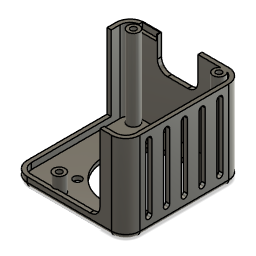
Fan Shroud (Autodesk Fusion 360 design; units mm, degrees)
Autodesk Fusion 360 part; units mm, degrees
sketch "Sketch1" plane through (0, 0, 0) normal (0, 1, 0) x (1, 0, 0)
  circle A0 centre (0, 0) radius 19
  circle A1 centre (-16, 16) radius 2
  circle A2 centre (16, 16) radius 2
  circle A3 centre (16, -16) radius 2
  circle A4 centre (-16, -16) radius 2
  line L0 (-26.4, 25.4) -> (15.2, 25.4)
  line L1 (20.2, 20.4) -> (20.2, -23.4)
  line L2 (15.2, -28.4) -> (-26.4, -28.4)
  line L3 (-31.4, -23.4) -> (-31.4, 20.4)
  line L4 (9.5, -30.4) -> (9.5, -28.4)
  line L5 (-31.4, 16) -> (-33.4, 16)
  arc A5 (15.2, -28.4) -> (20.2, -23.4) centre (15.2, -23.4) ccw
  arc A6 (20.2, 20.4) -> (15.2, 25.4) centre (15.2, 20.4) ccw
  arc A7 (-26.4, 25.4) -> (-31.4, 20.4) centre (-26.4, 20.4) ccw
  arc A8 (-31.4, -23.4) -> (-26.4, -28.4) centre (-26.4, -23.4) ccw
  line L6 (15.2, -30.4) -> (-26.4, -30.4)
  arc A9 (-33.4, -23.4) -> (-26.4, -30.4) centre (-26.4, -23.4) ccw
  line L7 (-33.4, -23.4) -> (-33.4, 20.4)
  arc A10 (-26.4, 27.4) -> (-33.4, 20.4) centre (-26.4, 20.4) ccw
  line L8 (-26.4, 27.4) -> (15.2, 27.4)
  arc A11 (22.2, 20.4) -> (15.2, 27.4) centre (15.2, 20.4) ccw
  line L9 (22.2, 20.4) -> (22.2, -23.4)
  arc A12 (15.2, -30.4) -> (22.2, -23.4) centre (15.2, -23.4) ccw
  dimension "d3" = 38
  dimension "d4" = 4
  dimension "d5" = 4
  dimension "d6" = 4
  dimension "d7" = 4
  dimension "d8" = 32
  dimension "d9" = 32
  dimension "d10" = 16
  dimension "d11" = 16
  dimension "d33" = 20.2
  dimension "d46" = 25.4
  dimension "d47" = 28.4
  dimension "d55" = 31.4
  dimension "d56" = 9.5
  dimension "d81" = 5
  dimension "d82" = 2
  dimension "d138" = 5
  dimension "d139" = 5
  dimension "d140" = 5
  dimension "d141" = 16
  constraint coincident A0.centre origin
  constraint vertical A1.centre A4.centre
  constraint horizontal A1.centre A2.centre
  constraint vertical A2.centre A3.centre
  constraint horizontal A3.centre A4.centre
  constraint horizontal L0
  constraint vertical L1
  constraint horizontal L2
  constraint vertical L3
  constraint coincident L2 L4.end
  constraint perpendicular L2 L4
  constraint coincident L3 L5.start
  constraint tangent L2 A5
  constraint tangent L1 A5
  constraint tangent L0 A6
  constraint tangent L1 A6
  constraint tangent L0 A7
  constraint tangent L3 A7
  constraint tangent L3 A8
  constraint tangent L2 A8
  constraint coincident L4.start L6
  constraint horizontal L5
  constraint coincident L5.end L7
  measures "d3" diameter of A0
  measures "d4" diameter of A1
  measures "d5" diameter of A2
  measures "d6" diameter of A3
  measures "d7" diameter of A4
  measures "d8" distance of A1.centre A4.centre
  measures "d9" distance of A3.centre A4.centre
  measures "d10" horizontal distance of A0.centre A4.centre
  measures "d11" vertical distance of A0.centre A4.centre
  measures "d33" distance of A0.centre L1
  measures "d46" distance of A0.centre L0
  measures "d47" distance of A0.centre L2
  measures "d55" distance of A0.centre L3
  measures "d56" distance of A0.centre L4
  measures "d81" radius of A8
  measures "d138" radius of A7
  measures "d139" radius of A6
  measures "d140" radius of A5
  measures "d141" distance of A0.centre L5
extrude "Extrude1" add sketch "Sketch1" along normal blind 2 contours L0 L1 L2 L3 A5 A6 A7 A8 makes body 1
sketch "Sketch2" plane through (0, 2, 0) normal (0, 1, 0) x (-1, 0, 0)
  circle A0 centre (-16, -16) radius 2
  circle A1 centre (0, 0) radius 19
  circle A2 centre (16, 16) radius 2
  circle A3 centre (-16, 16) radius 2
  circle A4 centre (16, -16) radius 2
  circle A5 centre (-14.75, -23) radius 1.4
  circle A6 centre (26.4, -22) radius 1.4
  circle A7 centre (15, 26) radius 1.4
  line L0 (31.4, -20.4) -> (31.4, 23.4)
  line L1 (26.4, 28.4) -> (-15.2, 28.4)
  line L2 (-20.2, 23.4) -> (-20.2, -20.4)
  line L3 (-15.2, -25.4) -> (26.4, -25.4)
  arc A8 (-15.2, 28.4) -> (-20.2, 23.4) centre (-15.2, 23.4) ccw
  arc A9 (-20.2, -20.4) -> (-15.2, -25.4) centre (-15.2, -20.4) ccw
  arc A10 (26.4, -25.4) -> (31.4, -20.4) centre (26.4, -20.4) ccw
  arc A11 (31.4, 23.4) -> (26.4, 28.4) centre (26.4, 23.4) ccw
  circle A12 centre (26.4, -22) radius 2.9
  circle A13 centre (-14.75, -23) radius 2.9
  circle A14 centre (15, 26) radius 2.9
  line L4 (20.2, -20.2) -> (-20.2, -20.2)
  line L5 (-20.2, -20.2) -> (-20.2, 20.2)
  line L6 (-20.2, 20.2) -> (20.2, 20.2)
  line L7 (20.2, 20.2) -> (20.2, -20.2)
  line L8 (20.2, -20.2) -> (-20.2, 20.2) construction
  line L9 (-20.2, -20.2) -> (20.2, 20.2) construction
  dimension "d14" = 2.8
  dimension "d16" = 23
  dimension "d17" = 2.8
  dimension "d19" = 22
  dimension "d26" = 2.8
  dimension "d57" = 26.4
  dimension "d58" = 14.75
  dimension "d88" = 1.5
  dimension "d89" = 1.5
  dimension "d90" = 1.5
  dimension "d91" = 40.4
  dimension "d92" = 40.4
  dimension "d142" = 48
  dimension "d143" = 11.4
  constraint horizontal L4
  constraint perpendicular L4 L5
  constraint parallel L4 L6
  constraint parallel L5 L7
  constraint coincident L8 A1.centre
  constraint coincident L9 A1.centre
  constraint coincident A1.centre origin
  measures "d14" diameter of A5
  measures "d16" vertical distance of A1.centre A5.centre
  measures "d17" diameter of A6
  measures "d19" vertical distance of A1.centre A6.centre
  measures "d26" diameter of A7
  measures "d57" horizontal distance of A1.centre A6.centre
  measures "d58" horizontal distance of A1.centre A5.centre
  measures "d91" distance of L5.end L6.end
  measures "d92" distance of L4.end L5.end
  measures "d142" vertical distance of A6.centre A7.centre
  measures "d143" horizontal distance of A6.centre A7.centre
extrude "Extrude2" add sketch "Sketch2" along normal blind 41.5 contours L3 A9 A13 | L3 A9 A13 L4 | A13 L4 bodies 1
extrude "Extrude3" add sketch "Sketch2" along normal blind 40 contours A12 bodies 1
extrude "Extrude4" add sketch "Sketch2" along normal blind 8.6 contours L1 A14 | L1 A14 bodies 1
extrude "Extrude6" add sketch "Sketch1" along normal blind 43.5 contours L0 L1 L2 L3 L4 L5 A5 A6 A7 L6 L7 A10 L8 A11 L9 A12 bodies 1
extrude "Extrude7" add sketch "Sketch1" along normal blind 5 separate body contours L2 L3 L4 L5 A8 L6 A9 L7 makes body 2
sketch "Sketch3" plane through (0, 0, -27.4) normal (0, 0, -1) x (-1, 0, 0)
  line L0 (-15.2, 0) -> (26.4, 0)
  line L1 (26.4, 0) -> (26.4, 43.5)
  line L2 (26.4, 43.5) -> (-15.2, 43.5)
  line L3 (-15.2, 43.5) -> (-15.2, 0)
  line L4 (-2, 43.5) -> (18, 43.5)
  line L5 (18, 43.5) -> (18, 31.5)
  line L6 (13, 26.5) -> (3, 26.5)
  line L7 (-2, 31.5) -> (-2, 43.5)
  arc A0 (13, 26.5) -> (18, 31.5) centre (13, 31.5) ccw
  arc A1 (-2, 31.5) -> (3, 26.5) centre (3, 31.5) ccw
  line L8 (-15.2, 0) -> (26.4, 0)
  line L9 (26.4, 0) -> (26.4, 43.5)
  line L10 (26.4, 43.5) -> (-15.2, 43.5)
  line L11 (-15.2, 43.5) -> (-15.2, 0)
  dimension "d67" = 17
  dimension "d68" = 5
  dimension "d144" = 2
  dimension "d145" = 20
  constraint horizontal L4
  constraint perpendicular L4 L5
  constraint parallel L4 L6
  constraint parallel L5 L7
  constraint coincident L2.end L4
  constraint tangent L5 A0
  constraint tangent L6 A0
  constraint tangent L6 A1
  constraint tangent L7 A1
  constraint equal A0 A1
  measures "d67" distance of L4 L6
  measures "d68" radius of A0
  measures "d144" distance of origin L7
  measures "d145" distance of L5 L7
extrude "Extrude8" cut sketch "Sketch3" against normal blind 2 contours L2 L4 L5 L6 L7 A0 A1 L10 bodies 1
combine "Combine1" operation add target body 2 tool bodies 1
fillet "Fillet1" radius 5 1 edges at (9.5, 5, 29.4) on bodies 2
fillet "Fillet2" radius 2.5 8 edges at (-31.3497, 0, 28.3497) (-5.6, 0, 30.4) (20.1497, 0, 28.3497) (22.2, 0, 1.5) (20.1497, 0, -25.3497) (-5.6, 0, -27.4) (-31.3497, 0, -25.3497) (-33.4, 0, 1.5) on bodies 2
sketch "Sketch14" plane through (0, 43.5, 0) normal (0, 1, 0) x (-1, 0, 0)
  line L0 (18, -25.4) -> (18, -27.4)
  line L1 (18, -27.4) -> (26.4, -27.4)
  arc A0 (26.4, -27.4) -> (33.4, -20.4) centre (26.4, -20.4) ccw
  line L2 (33.4, -20.4) -> (33.4, -16)
  line L3 (33.4, -16) -> (31.4, -16)
  line L4 (31.4, -16) -> (31.4, -20.4)
  arc A1 (26.4, -25.4) -> (31.4, -20.4) centre (26.4, -20.4) ccw
  line L5 (26.4, -25.4) -> (18, -25.4)
extrude "Extrude14" cut sketch "Sketch14" against normal blind 1.5 bodies 2
sketch "Sketch17" plane through (0, 42, 0) normal (0, 1, 0) x (-1, 0, 0)
  line L0 (26.4, -25.4) -> (18, -25.4)
  line L1 (18, -27.4) -> (26.4, -27.4)
  arc A0 (26.4, -27.4) -> (33.4, -20.4) centre (26.4, -20.4) ccw
  line L2 (33.4, -20.4) -> (33.4, -16)
  line L3 (33.4, -16) -> (31.4, -16)
  line L4 (31.4, -16) -> (31.4, -20.4)
  arc A1 (26.4, -25.4) -> (31.4, -20.4) centre (26.4, -20.4) ccw
  line L5 (18.4, -27) -> (27, -27)
  line L6 (27, -27) -> (27, -25.3639)
  line L7 (18.4, -25.3639) -> (18.4, -27)
  line L8 (18, -25.4) -> (18, -27.4)
  line L9 (19, -26.5) -> (27, -26.5)
  dimension "d133" = 8.6
  dimension "d134" = 0.4
  dimension "d162" = 0.4
  dimension "d163" = 8
  constraint horizontal L5
  constraint vertical L6
  constraint vertical L7
  constraint coincident A1 L6.end
  constraint perpendicular L7 L9
  measures "d133" distance of L5.start L5.end
  measures "d134" distance of L1 L5
  measures "d162" distance of L7 L8
  measures "d163" distance of L9.start L9.end
extrude "Extrude15" cut sketch "Sketch17" against normal blind 3 contours L0 A1 L5 L6 L7 bodies 2
sketch "Sketch19" plane through (22.2, 0, 0) normal (1, 0, 0) x (0, 0, -1)
  line L0 (-23.4, 2.5) -> (20.4, 2.5)
  line L1 (20.4, 2.5) -> (20.4, 43.5)
  line L2 (20.4, 43.5) -> (-23.4, 43.5)
  line L3 (-23.4, 43.5) -> (-23.4, 2.5)
  line L4 (-20.52, 6.88) -> (-20.52, 39.12)
  line L5 (-17.52, 39.12) -> (-17.52, 6.88)
  line L6 (-17.52, 5.88) -> (-20.52, 40.62) construction
  line L7 (-20.52, 5.88) -> (-17.52, 40.62) construction
  arc A0 (-19.02, 40.62) -> (-20.52, 39.12) centre (-19.02, 39.12) ccw
  arc A1 (-17.52, 39.12) -> (-19.02, 40.62) centre (-19.02, 39.12) ccw
  arc A2 (-19.0138, 5.38) -> (-17.52, 6.88) centre (-19.02, 6.88) ccw
  arc A3 (-20.52, 6.88) -> (-19.0138, 5.38) centre (-19.02, 6.88) ccw
  line L8 (-11.76, 5.88) -> (-8.76, 40.62) construction
  line L9 (-8.76, 39.12) -> (-8.76, 6.88)
  line L10 (-8.76, 5.88) -> (-11.76, 40.62) construction
  line L11 (-11.76, 6.88) -> (-11.76, 39.12)
  arc A4 (-10.26, 40.62) -> (-11.76, 39.12) centre (-10.26, 39.12) ccw
  arc A5 (-11.76, 6.88) -> (-10.2538, 5.38) centre (-10.26, 6.88) ccw
  arc A6 (-10.2538, 5.38) -> (-8.76, 6.88) centre (-10.26, 6.88) ccw
  arc A7 (-8.76, 39.12) -> (-10.26, 40.62) centre (-10.26, 39.12) ccw
  line L12 (-3, 5.88) -> (0, 40.62) construction
  line L13 (0, 39.12) -> (0, 6.88)
  line L14 (0, 5.88) -> (-3, 40.62) construction
  line L15 (-3, 6.88) -> (-3, 39.12)
  arc A8 (-1.5, 40.62) -> (-3, 39.12) centre (-1.5, 39.12) ccw
  arc A9 (-3, 6.88) -> (-1.4938, 5.38) centre (-1.5, 6.88) ccw
  arc A10 (-1.4938, 5.38) -> (0, 6.88) centre (-1.5, 6.88) ccw
  arc A11 (0, 39.12) -> (-1.5, 40.62) centre (-1.5, 39.12) ccw
  line L16 (5.76, 5.88) -> (8.76, 40.62) construction
  line L17 (8.76, 39.12) -> (8.76, 6.88)
  line L18 (8.76, 5.88) -> (5.76, 40.62) construction
  line L19 (5.76, 6.88) -> (5.76, 39.12)
  arc A12 (7.26, 40.62) -> (5.76, 39.12) centre (7.26, 39.12) ccw
  arc A13 (5.76, 6.88) -> (7.2662, 5.38) centre (7.26, 6.88) ccw
  arc A14 (7.2662, 5.38) -> (8.76, 6.88) centre (7.26, 6.88) ccw
  arc A15 (8.76, 39.12) -> (7.26, 40.62) centre (7.26, 39.12) ccw
  line L20 (14.52, 5.88) -> (17.52, 40.62) construction
  line L21 (17.52, 39.12) -> (17.52, 6.88)
  line L22 (17.52, 5.88) -> (14.52, 40.62) construction
  line L23 (14.52, 6.88) -> (14.52, 39.12)
  arc A16 (16.02, 40.62) -> (14.52, 39.12) centre (16.02, 39.12) ccw
  arc A17 (14.52, 6.88) -> (16.0262, 5.38) centre (16.02, 6.88) ccw
  arc A18 (16.0262, 5.38) -> (17.52, 6.88) centre (16.02, 6.88) ccw
  arc A19 (17.52, 39.12) -> (16.02, 40.62) centre (16.02, 39.12) ccw
  point P0 (-19.02, 23.25)
  point P1 (-10.26, 23.25)
  point P2 (-1.5, 23.25)
  point P3 (7.26, 23.25)
  point P4 (16.02, 23.25)
  dimension "d137" = 3
  dimension "d151" = 4.38
  dimension "d152" = 1.5
  dimension "d155" = 0
  dimension "d156" = 8.76
  dimension "d160" = 4.38
  dimension "d161" = 4.38
  constraint parallel L4 L5
  constraint coincident L6 P0
  constraint coincident L7 P0
  constraint coincident L6.end L4
  constraint tangent L4 A0
  constraint coincident L7.end L5
  constraint tangent L5 A1
  constraint equal A0 A1
  constraint coincident A0.start A1.end
  constraint coincident L6.start L5
  constraint tangent L5 A2
  constraint equal A0 A2
  constraint coincident L7.start L4
  constraint tangent L4 A3
  constraint equal A0 A3
  constraint coincident A2.start A3.end
  constraint coincident A2.centre A3.centre
  measures "d137" distance of L6.end L7.end
  measures "d151" distance of L3 P0
  measures "d152" radius of A0
  measures "d160" distance of L2 A0.centre
  measures "d161" distance of L0 A2.centre
extrude "Extrude16" cut sketch "Sketch19" against normal blind 2 contours L4 L5 A0 A1 A2 A3 | L9 L11 A4 A5 A6 A7 | L13 L15 A8 A9 A10 A11 | L17 L19 A12 A13 A14 A15 | L21 L23 A16 A17 A18 A19 bodies 2
equation "d10 = ( 32 / 2 ) * 1 mm"
equation "d11 = ( 32 / 2 ) * 1 mm"
equation "d33 = ( ( 40 / 2 ) * 1 mm ) + 0.2 mm"
equation "d46 = 23 mm + ( ( ( 2.8 / 2 ) * 1 mm ) + 1 * 1 mm )"
equation "d47 = 26 mm + ( ( ( 2.8 / 2 ) * 1 mm ) + 1 * 1 mm )"
equation "d48 = 41.5 mm + 2 mm"
equation "d55 = 21.4 mm + 10 mm"
equation "d56 = -5.5 mm + 15 mm"
equation "d91 = 40 mm + ( ( 0.2 * 2 ) * 1 mm )"
equation "d92 = 40 mm + ( ( 0.2 * 2 ) * 1 mm )"
equation "d141 = 22 mm - 6 mm"
equation "d142 = 42 mm + 6 mm"
equation "d151 = ( 8.76 / 2 ) * 1 mm"
equation "d152 = ( 3 / 2 ) * 1 mm"
equation "d156 = ( 43.8 / 5 ) * 1 mm"
equation "d160 = ( 8.76 / 2 ) * 1 mm"
equation "d161 = ( 8.76 / 2 ) * 1 mm"
